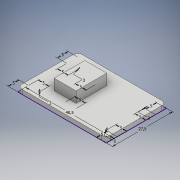
# Autodesk Inventor part: CASE ESP32 CAM - Tampa
Saved by Autodesk Inventor 2018 (Build 220112000, 112)
## iProperties
Created: 2022-03-15
Part Number: CASE ESP32 CAM - Tampa
Material: Genérico
Document SubType Name: Modeling
Designer: ADM
Density: 1 g/cm^3
Appearance: Padrão
Author: ADM
Autodesk Inventor part; units mm, degrees
ref_plane "YZ Plane" through (0, 0, 0) normal (1, 0, 0) x (0, 1, 0)
ref_plane "XZ Plane" through (0, 0, 0) normal (0, 1, 0) x (-1, 0, 0)
ref_plane "XY Plane" through (0, 0, 0) normal (0, 0, 1) x (1, 0, 0)
sketch "Esboço1" plane through (0, 0, 0) normal (0, 0, 1) x (1, 0, 0)
  line L0 (0, 0) -> (40.5, 0)
  line L1 (40.5, 0) -> (40.5, 27.5)
  line L2 (40.5, 27.5) -> (0, 27.5)
  line L3 (0, 27.5) -> (0, 0)
  line L4 (15, 20.75) -> (10, 20.75)
  line L5 (10, 20.75) -> (10, 6.75)
  line L6 (10, 6.75) -> (15, 6.75)
  line L7 (15, 6.75) -> (20, 6.75)
  line L8 (20, 6.75) -> (20, 20.75)
  line L9 (20, 20.75) -> (15, 20.75)
  line L10 (40.5, 27.5) -> (40.5, 22.5)
  line L11 (40.5, 22.5) -> (35.5, 22.5)
  line L12 (40.5, 0) -> (40.5, 5)
  line L13 (40.5, 5) -> (35.5, 5)
  line L14 (0, 0) -> (0, 5)
  line L15 (0, 5) -> (5, 5)
  line L16 (0, 27.5) -> (0, 22.5)
  line L17 (0, 22.5) -> (5, 22.5)
  circle A0 centre (5, 22.5) radius 1.5
  circle A1 centre (5, 5) radius 1.5
  circle A2 centre (35.5, 22.5) radius 1.5
  circle A3 centre (35.5, 5) radius 1.5
  dimension "d0" = 40.5
  dimension "d1" = 27.5
  dimension "d5" = 5
  dimension "d6" = 5
  dimension "d7" = 5
  dimension "d8" = 5
  dimension "d9" = 5
  dimension "d10" = 5
  dimension "d11" = 5
  dimension "d12" = 5
  dimension "d13" = 5
  dimension "d14" = 5
  dimension "d15" = 3
  dimension "d16" = 3
  dimension "d17" = 3
  dimension "d18" = 3
  constraints: 36 end point, 11 perpendicular, 6 point on line, 4 centre point, 4 coincident, 2 horizontal
  measures "d0" distance of L0.start L0.end
  measures "d1" distance of L0.end L1.end
  measures "d5" distance of L4.start L4.end
  measures "d6" distance of L6.end L7.end
  measures "d7" distance of L1.end L10.end
  measures "d8" distance of L10.end L11.end
  measures "d9" distance of L0.end L12.end
  measures "d10" distance of L12.end L13.end
  measures "d11" distance of L0.start L14.end
  measures "d12" distance of L14.end L15.end
  measures "d13" distance of L2.end L16.end
  measures "d14" distance of L16.end L17.end
  measures "d15" diameter of A0
  measures "d16" diameter of A1
  measures "d17" diameter of A2
  measures "d18" diameter of A3
extrude "Extrusão1" add sketch "Esboço1" along normal blind 2 contours L3 L2 L1 L0 | L9 L8 L7 L6 L5 L4
fillet "Arredondamento1" radius 2 4 edges at (0, 27.5, 1) (0, 0, 1) (40.5, 27.5, 1) (40.5, 0, 1)
extrude "Extrusão2" add sketch "Esboço1" along normal blind 7 contours L9 L8 L7 L6 L5 L4
extrude "Extrusão3" add sketch "Esboço1" along normal blind 2 contours A0 | A1 | A2 | A3
